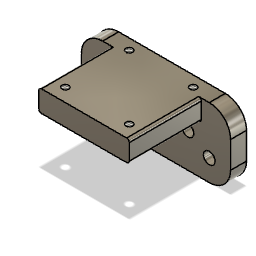
EX-0009723-000-XYZ-SLC-1730 z connector v9 (Autodesk Fusion 360 design; units mm, degrees)
Autodesk Fusion 360 part; units mm, degrees
sketch "Sketch2" plane through (0, 0, 0) normal (0, 0, 1) x (1, 0, 0)
  arc A0 (18.5, 20) -> (18, 20.5) centre (18, 20) ccw
  line L0 (18.5, 20) -> (18.5, 8.6168)
  arc A1 (18.5, 8.6168) -> (21.6842, 3.6281) centre (24, 8.6168) ccw
  arc A2 (20, -4) -> (21.6842, 3.6281) centre (20, 0) ccw
  line L1 (20, -4) -> (0, -4)
  arc A3 (-1.6842, 3.6281) -> (0, -4) centre (0, 0) ccw
  arc A4 (-1.6842, 3.6281) -> (1.5, 8.6168) centre (-4, 8.6168) ccw
  line L2 (1.5, 8.6168) -> (1.5, 20)
  arc A5 (2, 20.5) -> (1.5, 20) centre (2, 20) ccw
  line L3 (2, 20.5) -> (18, 20.5)
  circle A6 centre (20, 0) radius 1.1
  circle A7 centre (0, 0) radius 1.1
  line L4 (24, 9) -> (-4, 9)
  line L5 (-4, 0) -> (-4, 9)
  line L6 (24, 0) -> (24, 9)
  line L7 (1.5, 9) -> (1.5, 5)
  line L8 (1.5, 5) -> (18.5, 5)
  line L9 (18.5, 5) -> (18.5, 9)
  line L10 (10, -4) -> (10, 20.5) construction
  point P0 (4, 2.5)
  point P1 (16, 2.5)
  dimension "d2" = 9
  dimension "d6" = 4
  dimension "d20" = 12
  dimension "d21" = 2.5
  constraint horizontal L4
  constraint coincident A3 L5.start
  constraint coincident A2 L6.start
  constraint tangent A2 L6
  constraint tangent A3 L5
  constraint vertical L6
  constraint vertical L5
  constraint coincident L4 L7.start
  constraint coincident L2 L7.start
  constraint perpendicular L4 L7
  constraint perpendicular L0 L8
  constraint coincident L4 L9.end
  constraint coincident L0 L9.end
  constraint perpendicular L4 L9
  constraint midpoint L1 L10.start
  constraint midpoint L3 L10.end
  constraint horizontal P0 P1
  constraint symmetric L10 P0 P1
  measures "d2" distance of A3.centre L4
  measures "d6" distance of L4 L8
  measures "d20" distance of P0 P1
  measures "d21" distance of L8 P1
ref_plane "WorkPlane1" through (0, 9, 0) normal (0, 1, 0) x (0, 0, 1)
sketch "Sketch3" plane through (0, 9, 0) normal (0, 1, 0) x (1, 0, 0)
  circle A0 centre (4, -13.5) radius 0.625
  circle A1 centre (4, -13.5) radius 0.625
  circle A2 centre (16, -13.5) radius 0.625
  circle A3 centre (16, -13.5) radius 0.625
  circle A4 centre (16, -1.5) radius 0.625
  circle A5 centre (16, -1.5) radius 0.625
  circle A6 centre (4, -1.5) radius 0.625
  circle A7 centre (4, -1.5) radius 0.625
  dimension "d4" = 12
  dimension "d5" = 12
  measures "d4" distance of A2.centre A4.centre
  measures "d5" distance of A0.centre A2.centre
extrude "Extrude1" add sketch "Sketch2" along normal blind 2.5 and the other way blind 0.5 contours L0 A1 A2 L4 L6 L9 | L0 L2 L4 L7 L8 L9 | A1 A2 L1 A3 A4 L7 L8 L9 | A3 A4 L2 L4 L5 L7
extrude "Extrude2" add sketch "Sketch2" along normal blind 16 contours L0 L2 L4 L7 L8 L9
hole "Hole1" at (4, 9, 13.5) at (16, 9, 13.5) at (16, 9, 1.5) at (4, 9, 1.5) direction (0, -1, 0) diameter 1.271 depth 6.5 tip angle 118
thread "Thread1" "ISO Metric profile 1.6 M1.6x0.35 6H" thread offset 0 thread depth 10
fillet "Fillet1" radius 4 2 edges at (24, 9, 1) (-4, 9, 1)
fillet "Fillet1" radius 0.5 4 edges at (18.5, 9, 9.25) (1.5, 9, 9.25) (18.5, 5, 9.25) (1.5, 5, 9.25)
hole "Hole2" at (16, 2.5, 0) at (4, 2.5, 0) direction (0, 0, 1) diameter 2.2 depth 11 tip angle 118
hole "Hole3" at (16, 2.5, 0) at (4, 2.5, 0) direction (0, 0, -1) diameter 2.2 depth 11 tip angle 118
